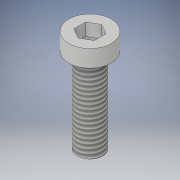
# Autodesk Inventor part: M6screw
Saved by Autodesk Inventor 2019 (Build 230136000, 136)
## iProperties
Created: 2020-01-03
Part Number: M6screw
Material: 一般
Document SubType Name: Modeling
Designer: user
Density: 1 g/cm^3
Appearance: 預設
Author: user
Autodesk Inventor part; units mm, degrees
ref_plane "YZ Plane" through (0, 0, 0) normal (1, 0, 0) x (0, 1, 0)
ref_plane "XZ Plane" through (0, 0, 0) normal (0, 1, 0) x (-1, 0, 0)
ref_plane "XY Plane" through (0, 0, 0) normal (0, 0, 1) x (1, 0, 0)
sketch "草圖1" plane through (0, 0, 0) normal (0, 1, 0) x (-1, 0, 0)
  circle A0 centre (0, 0) radius 3
  dimension "d0" = 6
  constraints: 1 centre point, 1 coincident
  measures "d0" diameter of A0
extrude "擠出1" add sketch "草圖1" along normal blind 20
thread "螺紋1" size "M6x1" class "6g" standard "ANSI Metric M Profile" full length
sketch "草圖2" plane through (0, 20, 0) normal (0, 1, 0) x (1, 0, 0)
  circle A0 centre (0, 0) radius 5
  dimension "d5" = 10
  constraints: 1 centre point, 1 coincident
  measures "d5" diameter of A0
extrude "擠出2" add sketch "草圖2" along normal blind 4
sketch "草圖3" plane through (0, 24, 0) normal (0, 1, 0) x (1, 0, 0)
  line L0 (0, 2.7818) -> (2.4091, 1.3909)
  line L1 (2.4091, 1.3909) -> (2.4091, -1.3909)
  line L2 (2.4091, -1.3909) -> (0, -2.7818)
  line L3 (0, -2.7818) -> (-2.4091, -1.3909)
  line L4 (-2.4091, -1.3909) -> (-2.4091, 1.3909)
  line L5 (-2.4091, 1.3909) -> (0, 2.7818)
  point P0 (0, 0)
  point P1 (0, 0)
  constraints: 12 end point, 1 coincident, 13 other
extrude "擠出3" cut sketch "草圖3" against normal blind 3
